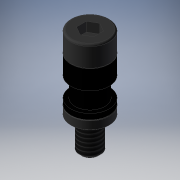
# Autodesk Inventor part: SCHUNK-5509536 Huelse MPG 40
Saved by Autodesk Inventor 2019 (Build 230136000, 136)
## iProperties
Created: 2022-08-29
Part Number: SCHUNK-5509536 Huelse MPG 40
Material: Generic
Catalog Web Link: www.cadenas.de
Description: Hülse-MPG
Vendor: SCHUNK
Document SubType Name: Modeling
Designer: psAdmin
Manufacturer: SCHUNK
Mass: 0.137802 g
Surface Area: 1.9535 cm^2
Volume: 0.137802 cm^3
Density: 1 g/cm^3
Appearance: PSOLRGB-175-175-175
Category: PARTsolutions
Company: SCHUNK
Title: SCHUNK-5509536 Huelse MPG 40
Author: Cadenas PARTsolutions
Comments: MPG
PSOL_IDENT_0: {$CADENAS_DATA/23d-libs/schunk/greifsysteme/greifmodule/greifmodule_pneumatisch/2_finger_parallelgre
PSOL_IDENT_1: ifer/2_finger_kleinteilegreifer/mpg/mpg_hul.prj},195 {VTYP=3D},{NB=SCHUNK-5509536 Huelse MPG 40},{LI
PSOL_IDENT_2: NA=SCHUNK-5509536 Huelse MPG 40},{NN=Hülse},{DATE=22.12.2021 07:17:05},{GEOMDATE=15.04.2020 08:38:32
PSOL_IDENT_3: },{VERSION=},{LINEID=40},{WBVAR=},{WBNUMERIC=}  {NB=SCHUNK-5509536 Huelse MPG 40},{LINA=SCHUNK-55095
PSOL_IDENT_4: 36 Huelse MPG 40},{KT=DUMMY},{IDNR=5509536},{TYP=MPG 40},{TYP1=7.000},{D1=4.500},{D2=2.500},{D3=3.50
PSOL_IDENT_5: 0},{H=5.300},{H1=2.300},{H2=2.300},{HZYL=2.400},{DZYL=4.500},{SW=2.000},{SWT=1.100},{DS=4.500},{HS=1
PSOL_IDENT_6: .000},{M1=2.500},{ML=10.000},{CNSCTN=84799070}
NB: SCHUNK-5509536 Huelse MPG 40
NN: Hülse
NT: MPG
NBSYN: SCHUNK-$IDNR. Huelse $TYP.
LINA: SCHUNK-5509536 Huelse MPG 40
CATALOG: SCHUNK
IDNR: 5509536
TYP: MPG 40
TYP1: 7
D1: 4.5
D2: 2.5
D3: 3.5
H: 5.3
H1: 2.3
H2: 2.3
HZYL: 2.4
DZYL: 4.5
SW: 2
SWT: 1.1
DS: 4.5
HS: 1
M1: 2.5
ML: 10
CNSCTN: 84799070
SUPPLIER: SCHUNK
ARTICLENO: SCHUNK-5509536 Huelse MPG 40
BOMINFO: SCHUNK-5509536 Huelse MPG 40
CREATOR: CADENAS GmbH
Autodesk Inventor part; units mm, degrees
sketch "Sketch_3" plane through (0, 0, 0) normal (1, 0, 0) x (0, 1, 0)
  line L0 (1, 0) -> (0, 0)
  line L1 (0, 0) -> (0, 2.2)
  line L2 (0, 2.2) -> (0.05, 2.25)
  line L3 (0.05, 2.25) -> (0.95, 2.25)
  line L4 (0.95, 2.25) -> (1, 2.2)
  line L5 (1, 2.2) -> (1, 0)
  line L6 (1, 0) -> (0, 0)
  constraints: 14 end point
revolve "Revolution1" add sketch "Sketch_3" angle 360 about axis through (0, 1, 0) along (0, 1, 0)
sketch "Sketch_9" plane through (0, 0, 0) normal (1, 0, 0) x (0, 1, 0)
  line L0 (-100, 0) -> (100, 0)
  line L1 (6.3, -1.25) -> (1, -1.25)
  line L2 (1, -1.25) -> (1, -2.2)
  line L3 (1, -2.2) -> (1.05, -2.25)
  line L4 (1.05, -2.25) -> (1.7, -2.25)
  line L5 (1.7, -2.25) -> (1.7, -1.75)
  line L6 (1.7, -1.75) -> (4, -1.75)
  line L7 (4, -1.75) -> (4, -2.25)
  line L8 (4, -2.25) -> (6.25, -2.25)
  line L9 (6.25, -2.25) -> (6.3, -2.2)
  line L10 (6.3, -2.2) -> (6.3, -1.25)
  constraints: 22 end point
revolve "Revolution2" add sketch "Sketch_9" angle 360 about axis through (0, -100, 0) along (0, -1, 0)
sketch "Sketch_6" plane through (0, 0, 0) normal (0, 0, 1) x (1, 0, 0)
  line L0 (0, -50) -> (0, 50)
  line L1 (0, 8.7) -> (2.05, 8.7)
  arc A0 (2.25, 8.5) -> (2.05, 8.7) centre (2.05, 8.5) ccw
  line L2 (2.25, 8.5) -> (2.25, 6.3)
  line L3 (2.25, 6.3) -> (0, 6.3)
  line L4 (0, 6.3) -> (0, 8.7)
  constraints: 10 end point, 2 point on circle, 1 centre point
revolve "Revolution3" add sketch "Sketch_6" angle 360 about axis through (0, -50, 0) along (0, -1, 0)
sketch "Sketch_7" plane through (0, 8.7, 0) normal (0, 1, 0) x (1, 0, 0)
  line L0 (-1, -0.5774) -> (0, -1.1547)
  line L1 (0, -1.1547) -> (1, -0.5774)
  line L2 (1, -0.5774) -> (1, 0.5774)
  line L3 (1, 0.5774) -> (0, 1.1547)
  line L4 (0, 1.1547) -> (-1, 0.5774)
  line L5 (-1, 0.5774) -> (-1, -0.5774)
  constraints: 12 end point
extrude "Extrusion1" cut sketch "Sketch_7" against normal blind 1.1
sketch "Sketch_10" plane through (0, 0, 0) normal (1, 0, 0) x (0, 1, 0)
  line L0 (-3.7, 0) -> (6.3, 0)
  line L1 (6.3, 0) -> (6.3, -1.25)
  line L2 (6.3, -1.25) -> (-3.424, -1.25)
  line L3 (-3.424, -1.25) -> (-3.7, -0.974)
  line L4 (-3.7, -0.974) -> (-3.7, 0)
  line L5 (-3.7, 0) -> (6.3, 0)
  constraints: 12 end point
revolve "Revolution4" add sketch "Sketch_10" angle 360 about axis through (0, -3.7, 0) along (0, -1, 0)
thread "Thread1" size "M2.5x0.45" class "6g" standard "ISO Metric profile" length 6.7723
ref_plane "AS_XY" through (0, 8.7, 0) normal (0, 1, 0) x (1, 0, 0)
ref_plane "AS_YZ" through (0, 8.7, 0) normal (1, 0, 0) x (0, 0, -1)
ref_plane "AS_ZX" through (0, 8.7, 0) normal (0, 0, -1) x (0, 1, 0)
ref_plane "hul_XY" through (0, 0, 0) normal (0, 1, 0) x (1, 0, 0)
ref_plane "hul_YZ" through (0, 0, 0) normal (1, 0, 0) x (0, 0, -1)
ref_plane "hul_ZX" through (0, 0, 0) normal (0, 0, -1) x (0, 1, 0)
ref_plane "s01_XY" through (0, 5.3, 0) normal (0, 1, 0) x (1, 0, 0)
ref_plane "s01_YZ" through (0, 5.3, 0) normal (1, 0, 0) x (0, 0, -1)
ref_plane "s01_ZX" through (0, 5.3, 0) normal (0, 0, -1) x (0, 1, 0)
body "Solid1"
